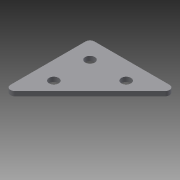
# Autodesk Inventor part: Camera Gusset Plat
Saved by Autodesk Inventor 2013 (Build 170138000, 138)
## iProperties
Created: 2013-01-24
Part Number: Camera Gusset Plat
Material: Generic
Document SubType Name: Modeling
Designer: actoennies
Density: 1 g/cm^3
Author: actoennies
Autodesk Inventor part; units mm, degrees
ref_plane "YZ Plane" through (0, 0, 0) normal (1, 0, 0) x (0, 1, 0)
ref_plane "XZ Plane" through (0, 0, 0) normal (0, 1, 0) x (-1, 0, 0)
ref_plane "XY Plane" through (0, 0, 0) normal (0, 0, 1) x (1, 0, 0)
sketch "Sketch1" plane through (0, 0, 0) normal (0, 1, 0) x (-1, 0, 0)
  circle A0 centre (-12.7, 12.7) radius 3.3782
  circle A1 centre (-12.7, 38.1) radius 3.3782
  circle A2 centre (-38.1, 12.7) radius 3.3782
  line L0 (0, 0) -> (0, -17.2047) construction
  line L1 (0, 3.175) -> (0, 55.8349)
  line L2 (-5.4201, 58.0799) -> (-58.0799, 5.4201)
  line L3 (-55.8349, 0) -> (-3.175, 0)
  arc A3 (-58.0799, 5.4201) -> (-55.8349, 0) centre (-55.8349, 3.175) ccw
  arc A4 (0, 55.8349) -> (-5.4201, 58.0799) centre (-3.175, 55.8349) ccw
  arc A5 (-3.175, 0) -> (0, 3.175) centre (-3.175, 3.175) ccw
  point P0 (0, -8.6024)
  point P1 (0, 63.5)
  point P2 (-63.5, 0)
  dimension "d3" = 6.7564
  dimension "d4" = 6.7564
  dimension "d5" = 6.7564
  dimension "d6" = 12.7
  dimension "d7" = 12.7
  dimension "d8" = 12.7
  dimension "d9" = 25.4
  dimension "d10" = 25.4
  dimension "d11" = 12.7
  dimension "d12" = 63.5
  dimension "d13" = 63.5
  dimension "d14" = 3.175
  constraints: 8 end point, 6 centre point, 6 point on circle, 6 point on line, 6 tangent, 2 equal radius, 1 collinear, 1 midpoint, 1 perpendicular, 1 vertical, 1 other
  measures "d3" diameter of A0
  measures "d4" diameter of A1
  measures "d5" diameter of A2
  measures "d6" horizontal distance of A0.centre L0.start
  measures "d7" distance from line of L0 A0.centre
  measures "d8" horizontal distance of L0.start A1.centre
  measures "d9" distance of A0.centre A1.centre
  measures "d10" distance of A2.centre A0.centre
  measures "d11" vertical distance of L0.start A2.centre
  measures "d12" distance of L0.start point (0, 63.5)
  measures "d13" distance of point (-63.5, 0) L0.start
  measures "d14" radius of A3
extrude "Extrusion1" add sketch "Sketch1" along normal blind 3.175
body "Solid1"
